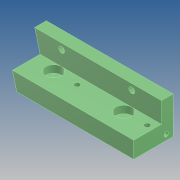
# Autodesk Inventor part: KB33-046-003-003 - Накладка на рычаг
Saved by Autodesk Inventor 2020 (Build 240168000, 168)
## iProperties
Created: 2021-06-25
Part Number: KB33-046-003-003 - Накладка на рычаг
Material: Пластик АБС
Document SubType Name: Modeling
Designer: Петров Иван
Mass: 34.5653 g
Surface Area: 104.659 cm^2
Volume: 32.6088 cm^3
Density: 1.06 g/cm^3
Appearance: Гладкий — темный травянисто-зеленый
Author: Петров Иван
Autodesk Inventor part; units mm, degrees
ref_plane "YZ Plane" through (0, 0, 0) normal (1, 0, 0) x (0, 1, 0)
ref_plane "XZ Plane" through (0, 0, 0) normal (0, 1, 0) x (-1, 0, 0)
ref_plane "XY Plane" through (0, 0, 0) normal (0, 0, 1) x (1, 0, 0)
sketch "Эскиз1" plane through (0, 0, 0) normal (0, 1, 0) x (-1, 0, 0)
  line L0 (-40, 13.5) -> (40, 13.5)
  line L1 (40, 13.5) -> (40, -13.5)
  line L2 (40, -13.5) -> (-40, -13.5)
  line L3 (-40, -13.5) -> (-40, 13.5)
  line L4 (-40, 13.5) -> (40, -13.5) construction
  line L5 (40, 13.5) -> (-40, -13.5) construction
  point P0 (0, 0)
  dimension "d0" = 80
  dimension "d1" = 27
  constraints: 12 end point, 2 midpoint, 2 parallel, 1 horizontal, 1 perpendicular
  measures "d0" distance of L1.end L2.end
  measures "d1" distance of L0.end L1.end
extrude "Выдавливание1" add sketch "Эскиз1" along normal blind 11.29
draft "НаклГрань1" angle -15 pull direction (0, 1, 0) faces at (-40, 7.5267, -4.5) fixed edges at (-40, 0, 0)
sketch "Эскиз3" plane through (0, 11.29, 0) normal (0, 1, 0) x (1, 0, 0)
  line L0 (40, 13.5) -> (-43.0251, 13.5) projected
  line L1 (40, -13.5) -> (40, 13.5) projected
  line L2 (-43.0251, 13.5) -> (40, 13.5)
  line L3 (40, 13.5) -> (40, 5.5)
  line L4 (40, 5.5) -> (-43.0251, 5.5)
  line L5 (-43.0251, 5.5) -> (-43.0251, 13.5)
  point P0 (0, 0)
  dimension "d8" = 8
  constraints: 8 end point, 2 parallel, 1 horizontal, 1 perpendicular, 1 point on line
  measures "d8" distance of L2.end L3.end
extrude "Выдавливание3" add sketch "Эскиз3" along normal blind 14
draft "НаклГрань2" angle -15 pull direction (0, 1, 0) faces at (-43.0251, 15.9567, -10.8333) fixed edges at (-43.0251, 11.29, -9.5)
sketch "Эскиз4" plane through (0, 11.29, 0) normal (0, 1, 0) x (1, 0, 0)
  circle A0 centre (19.7228, 0) radius 1.85 projected
  circle A1 centre (-12.2772, 0) radius 1.85 projected
  circle A2 centre (-28.2772, 0) radius 1.85 projected
  circle A3 centre (3.7228, 0) radius 1.85 projected
  circle A4 centre (35.7228, 0) radius 1.85 projected
  point P0 (0, 0)
extrude "Выдавливание4" cut sketch "Эскиз4" against normal blind 30.75 contours A0 | A1 | A2 | A4
sketch "Эскиз5" plane through (0, 11.29, 0) normal (0, 1, 0) x (1, 0, 0)
  circle A0 centre (-28.2772, 0) radius 1.85 projected
  circle A1 centre (-28.2772, 0) radius 5.5
  line L0 (40, 5.5) -> (-43.0251, 5.5) projected
  circle A2 centre (19.7228, 0) radius 1.85 projected
  circle A3 centre (19.7228, 0) radius 5.5
  point P0 (0, 0)
  constraints: 2 centre point, 2 coincident, 2 tangent
extrude "Выдавливание5" cut sketch "Эскиз5" against normal blind 5 contours A1 | A2 | A3
sketch "Эскиз6" plane through (40, 0, -13.5) normal (0, 0, -1) x (-1, 0, 0)
  line L0 (22.1272, 6.29) -> (18.4272, 6.29) projected
  line L1 (70.1272, 6.29) -> (66.4272, 6.29) projected
  line L2 (20.2772, 11.29) -> (68.2772, 11.29) projected
  line L3 (14.7772, 6.29) -> (25.7772, 6.29) projected
  line L4 (20.2772, 6.29) -> (20.2772, 21.29) construction
  circle A0 centre (20.2772, 21.29) radius 2
  line L5 (68.2772, 6.29) -> (68.2772, 21.29) construction
  circle A1 centre (68.2772, 21.29) radius 2
  point P0 (40, 0)
  dimension "d16" = 10
  dimension "d17" = 4
  dimension "d18" = 4
  constraints: 4 end point, 2 centre point, 2 coincident, 2 midpoint, 2 vertical, 1 horizontal alignment
  measures "d16" distance from line of L2 L4.end
  measures "d17" diameter of A0
  measures "d18" diameter of A1
extrude "Выдавливание6" cut sketch "Эскиз6" against normal blind 30.75
ref_plane "РабПлоскость1" through (35, 0, 13.5) normal (1, 0, 0) x (0, 0, -1)
sketch "Эскиз7" plane through (35, 0, 13.5) normal (1, 0, 0) x (0, 0, -1)
  line L0 (27, 0) -> (0, 0) projected
  line L1 (22.3954, 0) -> (19.2454, 1.8187)
  line L2 (19.2454, 1.8187) -> (19.2454, 5.456)
  line L3 (19.2454, 5.456) -> (22.3954, 7.2746)
  line L4 (22.3954, 7.2746) -> (25.5454, 5.456)
  line L5 (25.5454, 5.456) -> (25.5454, 1.8187)
  line L6 (25.5454, 1.8187) -> (22.3954, 0)
  line L7 (27, 0) -> (27, 25.29) projected
  line L8 (25.5454, 1.8187) -> (25.5454, 0)
  line L9 (19.2454, 1.8187) -> (19.2454, 0)
  point P0 (13.5, 0)
  point P1 (22.3954, 3.6373)
  dimension "d22" = 6.3
  constraints: 16 end point, 3 point on line, 2 perpendicular, 1 parallel, 13 other
  measures "d22" distance between parallel lines of L2 L5
extrude "Выдавливание7" cut sketch "Эскиз7" along normal mid plane 5
sketch "Эскиз9" plane through (40, 0, 13.5) normal (1, 0, 0) x (0, 0, -1)
  line L0 (27, 0) -> (0, 0)
  line L1 (22.3954, 0) -> (19.2454, 1.8187)
  line L2 (19.2454, 1.8187) -> (19.2454, 5.456)
  line L3 (19.2454, 5.456) -> (22.3954, 7.2746)
  line L4 (22.3954, 7.2746) -> (25.5454, 5.456)
  line L5 (25.5454, 5.456) -> (25.5454, 1.8187)
  line L6 (25.5454, 1.8187) -> (22.3954, 0)
  line L7 (27, 0) -> (27, 21.29)
  line L8 (25.5454, 1.8187) -> (25.5454, 0)
  line L9 (19.2454, 1.8187) -> (19.2454, 0)
  circle A0 centre (22.3954, 3.6373) radius 1.5
  point P0 (13.5, 0)
  point P1 (13.5, 0)
  dimension "d27" = 6.3
  dimension "d28" = 3
  constraints: 20 end point, 3 point on line, 2 perpendicular, 1 centre point, 1 coincident, 1 parallel, 13 other
  measures "d27" distance between parallel lines of L2 L5
  measures "d28" diameter of A0
extrude "Выдавливание8" cut sketch "Эскиз9" against normal blind 5 contours A0
equation "\"d18\" = d17"
